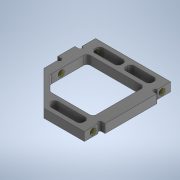
# Autodesk Inventor part: ForeArm_diagonal
Saved by Autodesk Inventor 2020 (Build 240168000, 168)
## iProperties
Part Number: ForeArm_diagonal
Material: アセタール樹脂、黒
Document SubType Name: Modeling
Designer: Masato Kubotera
Density: 1.425 g/cm^3
Appearance: 滑らか - 黒
Description: POM T5
Mass: 5.75609 g
Surface Area: 39.6633 cm^2
Volume: 4.03936 cm^3
Author: Masato Kubotera
Autodesk Inventor part; units mm, degrees
ref_plane "YZ Plane" through (0, 0, 0) normal (1, 0, 0) x (0, 1, 0)
ref_plane "XZ Plane" through (0, 0, 0) normal (0, 1, 0) x (-1, 0, 0)
ref_plane "XY Plane" through (0, 0, 0) normal (0, 0, 1) x (1, 0, 0)
derived "ForeArm_outside_frame.ipt"
sketch "スケッチ1" plane through (0, 0, 0) normal (0, 1, 0) x (-1, 0, 0)
  circle A0 centre (0, 0) radius 5.05
  line L0 (-8.5, 0) -> (8.5, 0) construction
  circle A1 centre (-8.5, 0) radius 1.35
  circle A2 centre (-6.0104, -6.0104) radius 1.35
  circle A3 centre (0, -8.5) radius 1.35
  circle A4 centre (6.0104, -6.0104) radius 1.35
  circle A5 centre (0, -145.8097) radius 16 construction
  line L1 (0, 0) -> (0, -145.8097) construction
  arc A6 (-20.3699, -115.9088) -> (20.3699, -115.9088) centre (0, -145.8097) ccw
  circle A7 centre (-8.5, 0) radius 2.4 construction
  line L2 (-16, 31) -> (16, 31) construction
  line L3 (16, 31) -> (16, -12) construction
  line L4 (16, -12) -> (-16, -12) construction
  line L5 (-16, -12) -> (-16, 31) construction
  line L6 (-16, 31) -> (16, -12) construction
  line L7 (16, 31) -> (-16, -12) construction
  arc A8 (-16, 0) -> (-10.583, -12) centre (0, 0) ccw construction
  arc A9 (10.583, -12) -> (16, 0) centre (0, 0) ccw construction
  line L8 (-16, -107.6443) -> (-16, 0)
  line L9 (16, -107.6443) -> (16, 0)
  circle A10 centre (0, -82.5) radius 1.6
  line L10 (0, -145.8097) -> (-25.5832, -120.2265) construction
  circle A11 centre (-22.7548, -123.055) radius 4 construction
  circle A12 centre (-22.7548, -123.055) radius 1.6
  circle A13 centre (-22.7548, -168.5645) radius 1.6
  circle A14 centre (22.7548, -168.5645) radius 1.6
  circle A15 centre (22.7548, -123.055) radius 1.6
  line L11 (30.6064, -21.0119) -> (2.8936, -37.0119) construction
  line L12 (2.8936, -37.0119) -> (-18.6064, 0.2272) construction
  line L13 (-18.6064, 0.2272) -> (9.1064, 16.2272) construction
  line L14 (9.1064, 16.2272) -> (30.6064, -21.0119) construction
  line L15 (30.6064, -21.0119) -> (-18.6064, 0.2272) construction
  line L16 (2.8936, -37.0119) -> (9.1064, 16.2272) construction
  line L17 (16.75, -29.0119) -> (-4.75, 8.2272) construction
  circle A16 centre (0, -42.5) radius 1.6
  line L18 (-2.5, -47.5) -> (2.5, -47.5) construction
  line L19 (2.5, -47.5) -> (2.5, -57.5) construction
  line L20 (2.5, -57.5) -> (-2.5, -57.5) construction
  line L21 (-2.5, -57.5) -> (-2.5, -47.5) construction
  line L22 (-2.5, -47.5) -> (2.5, -57.5) construction
  line L23 (2.5, -47.5) -> (-2.5, -57.5) construction
  line L24 (-2.5, -52.5) -> (2.5, -52.5) construction
  circle A17 centre (0, -62.5) radius 1.6
  line L25 (2.8936, -37.0119) -> (49.2811, -117.3573) construction
  line L26 (0, -145.8097) -> (49.2811, -117.3573) construction
  line L27 (-2.5, -47.5) -> (2.5, -47.5) construction
  line L28 (2.5, -47.5) -> (2.5, -77.5) construction
  line L29 (2.5, -77.5) -> (-2.5, -77.5) construction
  line L30 (-2.5, -77.5) -> (-2.5, -47.5) construction
  line L31 (-2.5, -47.5) -> (2.5, -77.5) construction
  line L32 (2.5, -47.5) -> (-2.5, -77.5) construction
  line L33 (-2.55, -47.45) -> (2.55, -47.45)
  line L34 (2.55, -47.45) -> (2.55, -77.55)
  line L35 (2.55, -77.55) -> (-2.55, -77.55)
  line L36 (-2.55, -77.55) -> (-2.55, -47.45)
  line L37 (-2.55, -47.45) -> (2.55, -77.55) construction
  line L38 (2.55, -47.45) -> (-2.55, -77.55) construction
  arc A18 (-1.0651, -47.45) -> (-2.55, -48.9349) centre (-1.8075, -48.1925) ccw
  arc A19 (2.55, -48.9349) -> (1.0651, -47.45) centre (1.8075, -48.1925) ccw
  line L39 (-2.5, -62.5) -> (2.5, -62.5) construction
  arc A20 (-2.55, -76.0651) -> (-1.0651, -77.55) centre (-1.8075, -76.8075) ccw
  arc A21 (1.0651, -77.55) -> (2.55, -76.0651) centre (1.8075, -76.8075) ccw
  arc A22 (16, 0) -> (8.0571, 13.8233) centre (0, 0) ccw
  circle A23 centre (0, -145.8097) radius 28.1801
  line L40 (-5.05, 0) -> (-5.05, 12.0954)
  line L41 (5.05, 0) -> (5.05, 12.0954)
  circle A24 centre (8.5, 0) radius 1.35
  arc A25 (-8.0571, 13.8233) -> (-16, 0) centre (0, 0) ccw
  arc A26 (-5.05, 12.0954) -> (-8.0571, 13.8233) centre (-7.05, 12.0954) ccw
  arc A27 (8.0571, 13.8233) -> (5.05, 12.0954) centre (7.05, 12.0954) ccw
  arc A28 (-20.3699, -115.9088) -> (-16, -107.6443) centre (-26, -107.6443) ccw
  arc A29 (16, -107.6443) -> (20.3699, -115.9088) centre (26, -107.6443) ccw
  point P0 (0, 9.5)
  point P1 (0, 9.5)
  point P2 (-16, -113.3598)
  point P3 (16, -113.3598)
  point P4 (6, -10.3923)
  point P5 (0, -52.5)
  point P6 (0, -62.5)
  point P7 (0, -181.9899)
  point P8 (-5.05, 15.1821)
  point P9 (5.05, 15.1821)
  point P10 (1.0651, -77.55)
  point P11 (-1.0651, -77.55)
  point P12 (-2.55, -76.0651)
  point P13 (2.55, -48.9349)
  point P14 (2.55, -76.0651)
  point P15 (5.05, 9.6596)
  point P16 (5.05, 0)
  dimension "d4" = 30
  dimension "d5" = 10
  dimension "d6" = 20
  dimension "d7" = 40
  dimension "d8" = 5
  measures "d4" distance of L28.end L18.end
  measures "d5" distance of L20.end L18.start
  measures "d6" distance of A17.centre A16.centre
  measures "d7" distance of A10.centre A16.centre
  measures "d8" distance of L27.start L27.end
sketch "スケッチ2" plane through (0, 0, 0) normal (1, 0, 0) x (0, 1, 0)
  line L0 (0, -37.5) -> (-43.5, -37.5)
  line L1 (0, -37.5) -> (0, -45.4)
  line L2 (0, -47.5) -> (2, -47.5)
  line L3 (2, -47.5) -> (2, -77.5)
  line L4 (2, -77.5) -> (0, -77.5)
  line L5 (0, -79.6) -> (0, -87.5)
  line L6 (0, -87.5) -> (-23.5, -87.5)
  line L7 (-43.5, -37.5) -> (-43.5, -45.4)
  line L8 (-43.5, -47.5) -> (-45.5, -47.5)
  line L9 (-45.5, -47.5) -> (-45.5, -57.5)
  line L10 (-45.5, -57.5) -> (-43.5, -57.5)
  line L11 (-43.5, -59.6) -> (-43.5, -67.5)
  line L12 (-43.5, -67.5) -> (-23.5, -87.5)
  line L13 (2, -62.5) -> (0, -62.5) construction
  arc A0 (0, -45.4) -> (0, -47.5) centre (0, -46.45) ccw
  line L14 (-45.5, -52.5) -> (-43.5, -52.5) construction
  arc A1 (0, -77.5) -> (0, -79.6) centre (0, -78.55) ccw
  arc A2 (-43.5, -47.5) -> (-43.5, -45.4) centre (-43.5, -46.45) ccw
  arc A3 (-43.5, -59.6) -> (-43.5, -57.5) centre (-43.5, -58.55) ccw
  line L15 (0, -42.5) -> (-5, -42.5) construction
  line L16 (0, -82.5) -> (-5, -82.5) construction
  line L17 (-7, -40) -> (-18.5, -40)
  line L18 (-20.5, -42) -> (-20.5, -43)
  line L19 (-18.5, -45) -> (-7, -45)
  line L20 (-5, -43) -> (-5, -42)
  line L21 (-5, -40) -> (-20.5, -45) construction
  line L22 (-20.5, -40) -> (-5, -45) construction
  line L23 (-7, -47.5) -> (-36.5, -47.5)
  line L24 (-5, -82) -> (-5, -83)
  line L25 (-7, -85) -> (-21.636, -85)
  line L26 (-23.0503, -84.4142) -> (-24.0503, -83.4142)
  line L27 (-22.636, -80) -> (-7, -80)
  line L28 (-38.5, -49.5) -> (-38.5, -68.136)
  line L29 (-5, -75.5) -> (-5, -49.5)
  line L30 (-7, -77.5) -> (-29.136, -77.5)
  line L31 (-30.5503, -76.9142) -> (-37.9142, -69.5503)
  arc A4 (-22.636, -80) -> (-24.0503, -83.4142) centre (-22.636, -82) ccw
  arc A5 (-23.0503, -84.4142) -> (-21.636, -85) centre (-21.636, -83) ccw
  arc A6 (-7, -85) -> (-5, -83) centre (-7, -83) ccw
  arc A7 (-5, -82) -> (-7, -80) centre (-7, -82) ccw
  arc A8 (-36.5, -47.5) -> (-38.5, -49.5) centre (-36.5, -49.5) ccw
  arc A9 (-5, -49.5) -> (-7, -47.5) centre (-7, -49.5) ccw
  arc A10 (-18.5, -40) -> (-20.5, -42) centre (-18.5, -42) ccw
  arc A11 (-20.5, -43) -> (-18.5, -45) centre (-18.5, -43) ccw
  arc A12 (-7, -45) -> (-5, -43) centre (-7, -43) ccw
  arc A13 (-5, -42) -> (-7, -40) centre (-7, -42) ccw
  line L32 (-21.75, -37.5) -> (-21.75, -87.5) construction
  line L33 (-23, -42) -> (-23, -43)
  arc A14 (-23, -42) -> (-25, -40) centre (-25, -42) ccw
  arc A15 (-25, -45) -> (-23, -43) centre (-25, -43) ccw
  arc A16 (-38.5, -43) -> (-36.5, -45) centre (-36.5, -43) ccw
  arc A17 (-36.5, -40) -> (-38.5, -42) centre (-36.5, -42) ccw
  line L34 (-36.5, -40) -> (-25, -40)
  line L35 (-38.5, -43) -> (-38.5, -42)
  line L36 (-25, -45) -> (-36.5, -45)
  arc A18 (-38.5, -68.136) -> (-37.9142, -69.5503) centre (-36.5, -68.136) ccw
  arc A19 (-30.5503, -76.9142) -> (-29.136, -77.5) centre (-29.136, -75.5) ccw
  arc A20 (-7, -77.5) -> (-5, -75.5) centre (-7, -75.5) ccw
  point P0 (0, 0)
  point P1 (0, -57.5)
  point P2 (0, -57.5)
  point P3 (0, -57.5)
  point P4 (0, -52.5)
  point P5 (0, -52.5)
  point P6 (0, -52.5)
  point P7 (0, -62.5)
  point P8 (-12.75, -42.5)
  point P9 (-5, -47.5)
  point P10 (-38.5, -47.5)
  point P11 (-5, -85)
  point P12 (-5, -80)
  point P13 (-22.4645, -85)
  point P14 (-38.5, -68.9645)
  dimension "d1" = 43.5
  dimension "d2" = 2
  dimension "d3" = 2
  dimension "d9" = 30
  dimension "d11" = 1.05
  dimension "d12" = 10
  dimension "d13" = 10
  dimension "d14" = 1.05
  dimension "d15" = 5
  dimension "d16" = 40
  dimension "d17" = 2.5
  dimension "d18" = 2.5
  dimension "d38" = 2.5
  dimension "d40" = 2.5
  dimension "d41" = 2
  dimension "d44" = 135
  dimension "d46" = 2
  dimension "d47" = 2
  dimension "d48" = 2.5
  constraints: 75 end point, 42 point on circle, 33 point on line, 28 tangent, 21 centre point, 21 symmetric about line, 10 equal radius, 9 perpendicular, 7 horizontal, 6 midpoint, 5 parallel, 4 collinear, 3 vertical, 1 coincident, 6 other
  measures "d1" distance of L0.start L0.end
  measures "d2" distance of L8.start L8.end
  measures "d3" distance of L2.start L2.end
  measures "d9" distance of L2.end L3.end
  measures "d11" radius of A0
  measures "d12" vertical distance of L0.start L2.end
  measures "d13" vertical distance of L5.end L3.end
  measures "d14" radius of A2
  measures "d15" distance of L15.end L15.start
  measures "d16" distance of L16.start L15.start
  measures "d17" vertical distance of L0.start L21.start
  measures "d18" distance between parallel lines of L12 L26
  measures "d38" distance between parallel lines of L23 L19
  measures "d40" distance between parallel lines of L27 L30
  measures "d41" radius of A4
  measures "d44" angle of L11 L12
  measures "d46" radius of A8
  measures "d47" radius of A18
  measures "d48" distance between parallel lines of L18 L33
extrude "押し出し1" add sketch "スケッチ2" along normal mid plane 5
hole "穴1" at (0, 0, -42.5) at (0, 0, -82.5) direction (0, -1, 0) diameter 3.4587 depth 6 thread size "M4x0.5" class "6H" standard "ISO Metric profile"
sketch "スケッチ3" plane through (-2.5, -43.5, -45.4) normal (0, -1, 0) x (1, 0, 0)
  line L0 (5, -7.1) -> (0, -7.1)
  line L1 (5, -2.1) -> (5, -12.1) projected
  line L2 (0, -12.1) -> (0, -2.1) projected
  arc A0 (0.8445, 3.4) -> (0.8445, 2.4) centre (2.5, 2.9) ccw projected
  point P0 (2.5, 45.4)
  point P1 (2.5, -17.1)
  constraints: 2 end point, 2 midpoint, 1 coincident, 1 horizontal, 1 symmetric about line
hole "穴2" at (0, -43.5, -42.5) at (0, -43.5, -62.5) direction (0, 1, 0) diameter 3.4587 depth 6 thread size "M4x0.5" class "6H" standard "ISO Metric profile"
equation "\"d9\" = d4"
equation "\"d14\" = d11"
equation "\"d16\" = d7"
equation "\"d20\" = d15"
